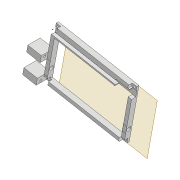
# Autodesk Inventor part: Rail_stage_y_v1
Saved by Autodesk Inventor 2020 (Build 240168000, 168)
## iProperties
Created: 2022-01-11
Part Number: Rail_stage_y_v1
Material: Generic
Document SubType Name: Modeling
Designer: CDT
Density: 1 g/cm^3
Appearance: Default
Author: CDT
Autodesk Inventor part; units mm, degrees
ref_plane "YZ Plane" through (0, 0, 0) normal (1, 0, 0) x (0, 1, 0)
ref_plane "XZ Plane" through (0, 0, 0) normal (0, 1, 0) x (-1, 0, 0)
ref_plane "XY Plane" through (0, 0, 0) normal (0, 0, 1) x (1, 0, 0)
ref_plane "Work Plane1" through (34.4543, -4.3418, 1.4) normal (0, 0, 1) x (0.9837071, -0.1797788, 0)
sketch "Sketch1" plane through (34.4543, -4.3418, 1.4) normal (0, 0, 1) x (0.9837071, -0.1797788, 0)
  line L0 (38.644, 42.2221) -> (-81.356, 42.2221)
  line L1 (-81.356, 42.2221) -> (-81.356, -37.7779)
  line L2 (-81.356, -37.7779) -> (38.644, -37.7779)
  line L3 (38.644, -37.7779) -> (38.644, 42.2221)
  circle A0 centre (35.644, 39.2221) radius 1.5
  circle A1 centre (35.644, -34.7779) radius 1.5
  circle A2 centre (-78.356, 39.2221) radius 1.5
  circle A3 centre (-78.356, -34.7779) radius 1.5
  line L4 (-76.356, 37.2221) -> (33.644, 37.2221)
  line L5 (33.644, 37.2221) -> (33.644, -32.7779)
  line L6 (33.644, -32.7779) -> (-76.356, -32.7779)
  line L7 (-76.356, -32.7779) -> (-76.356, 37.2221)
  line L8 (33.644, -11.7779) -> (32.644, -11.7779)
  line L9 (32.644, -11.7779) -> (32.644, -21.7779)
  line L10 (32.644, -21.7779) -> (33.644, -21.7779)
  line L11 (33.644, -21.7779) -> (33.644, -11.7779)
  point P0 (-34.6735, -1.9231)
  point P1 (33.644, -21.7779)
  dimension "d0" = 120
  dimension "d1" = 80
  dimension "d2" = 3
  dimension "d3" = 3
  dimension "d4" = 3
  dimension "d5" = 3
  dimension "d6" = 3
  dimension "d7" = 3
  dimension "d8" = 3
  dimension "d9" = 3
  dimension "d10" = 3
  dimension "d11" = 3
  dimension "d12" = 3
  dimension "d13" = 3
  dimension "d16" = 5
  dimension "d64" = 11
  dimension "d65" = 1
  dimension "d66" = 10
  constraints: 24 end point, 6 parallel, 4 centre point, 3 perpendicular, 2 horizontal, 1 point on line, 3 other
  measures "d0" distance of L2.end L1.end
  measures "d1" distance of L1.end L0.end
  measures "d2" diameter of A0
  measures "d3" diameter of A1
  measures "d4" diameter of A2
  measures "d5" diameter of A3
  measures "d6" distance from line of L0 A0.centre
  measures "d7" distance from line of L3 A0.centre
  measures "d8" distance from line of L2 A1.centre
  measures "d9" distance from line of L3 A1.centre
  measures "d10" distance from line of L1 A2.centre
  measures "d11" distance from line of L0 A2.centre
  measures "d12" distance from line of L1 A3.centre
  measures "d13" distance from line of L2 A3.centre
  measures "d16" distance between parallel lines of L0 L4
  measures "d64" distance between parallel lines of L6 L10
  measures "d65" distance between parallel lines of L5 L9
  measures "d66" distance between parallel lines of L10 L8
extrude "Extrusion1" add sketch "Sketch1" along normal blind 8 contours L3 L2 L1 L0 | L5 L10 L9 L8
sketch "Sketch3" plane through (34.4543, -4.3418, 9.4) normal (0, 0, 1) x (0.9837071, -0.1797788, 0)
  circle A0 centre (35.644, 39.2221) radius 1.5 projected
  circle A1 centre (35.644, -34.7779) radius 1.5 projected
  circle A2 centre (-78.356, 39.2221) radius 1.5 projected
  circle A3 centre (-78.356, -34.7779) radius 1.5 projected
  point P0 (-34.6735, -1.9231)
  point P1 (35.644, 39.2221)
  point P2 (35.644, -34.7779)
  point P3 (-78.356, 39.2221)
  point P4 (-78.356, -34.7779)
  constraints: 4 coincident
hole "Hole1" at (76.5689, 27.8333, 9.4) at (63.2653, -44.9611, 9.4) at (-35.5737, 48.328, 9.4) at (-48.8773, -24.4663, 9.4) direction (0, 0, -1) diameter 3.1 depth 8 tip angle 118 counterbore diameter 10 counterbore depth 5
sketch "Sketch6" plane through (34.4543, -4.3418, 1.4) normal (0, 0, -1) x (-0.9837071, 0.1797788, 0)
  line L0 (76.356, 37.2221) -> (-33.644, 37.2221) projected
  line L1 (76.356, 37.2221) -> (-33.644, 37.2221)
  line L2 (-33.644, 37.2221) -> (-33.644, 27.2221)
  line L3 (-33.644, 27.2221) -> (76.356, 27.2221)
  line L4 (76.356, 27.2221) -> (76.356, 37.2221)
  point P0 (34.6735, -1.9231)
  point P1 (-33.644, 37.2221)
  dimension "d43" = 110
  dimension "d44" = 10
  constraints: 8 end point, 2 parallel, 1 horizontal, 1 perpendicular
  measures "d43" distance of L3.end L2.end
  measures "d44" distance of L2.end L1.end
extrude "Extrusion5" add sketch "Sketch6" against normal up to surface (8 mm away)
sketch "Sketch7" plane through (34.4543, -4.3418, 9.4) normal (0, 0, 1) x (0.9837071, -0.1797788, 0)
  line L0 (38.644, 35.2221) -> (-81.356, 35.2221)
  line L1 (-81.356, 35.2221) -> (-81.356, 29.2221)
  line L2 (-81.356, 29.2221) -> (38.644, 29.2221)
  line L3 (38.644, 29.2221) -> (38.644, 35.2221)
  line L4 (31.644, 42.2221) -> (-74.356, 42.2221) projected
  line L5 (-81.356, 35.2221) -> (-81.356, -30.7779) projected
  line L6 (38.644, -30.7779) -> (38.644, 35.2221) projected
  point P0 (-34.6735, -1.9231)
  point P1 (38.644, 42.2221)
  point P2 (35.644, 42.2221)
  point P3 (-81.356, 42.2221)
  point P4 (-81.356, 39.2221)
  point P5 (38.644, -37.7779)
  point P6 (38.644, -34.7779)
  point P7 (-81.356, -37.7779)
  dimension "d47" = 6
  dimension "d48" = 7
  dimension "d49" = 0
  dimension "d50" = 0
  constraints: 8 end point, 2 parallel, 1 horizontal, 1 perpendicular
  measures "d47" distance of L1.end L0.end
  measures "d48" distance between parallel lines of L4 L0
  measures "d49" distance between parallel lines of L5 L1
  measures "d50" distance between parallel lines of L6 L3
extrude "Extrusion6" cut sketch "Sketch7" against normal blind 6 draft 10
sketch "Sketch8" plane through (65.6771, -48.4515, 1.4) normal (0.9837071, -0.1797788, 0) x (0, 0, -1)
  line L0 (-2, 74.5) -> (-9, 74.5)
  line L1 (-9, 74.5) -> (-9, 64.5)
  line L2 (-9, 64.5) -> (-2, 64.5)
  line L3 (-2, 64.5) -> (-2, 74.5)
  line L4 (0, 80) -> (-3, 80) projected
  line L5 (-2, 74.058) -> (-2, 65.942) projected
  point P0 (1.4, 35.8548)
  point P1 (-8, 80)
  dimension "d53" = 7
  dimension "d54" = 10
  dimension "d55" = 5.5
  dimension "d56" = 0
  constraints: 8 end point, 2 parallel, 1 horizontal, 1 perpendicular
  measures "d53" distance of L2.end L1.end
  measures "d54" distance of L1.end L0.end
  measures "d55" distance between parallel lines of L4 L0
  measures "d56" distance between parallel lines of L5 L3
extrude "Extrusion7" cut sketch "Sketch8" against normal blind 25
sketch "Sketch10" plane through (34.4543, -4.3418, 1.4) normal (0, 0, -1) x (-0.9837071, 0.1797788, 0)
  line L0 (81.356, 4.2221) -> (101.356, 4.2221)
  line L1 (101.356, 4.2221) -> (101.356, -5.7779)
  line L2 (101.356, -5.7779) -> (81.356, -5.7779)
  line L3 (81.356, -5.7779) -> (81.356, 4.2221)
  line L4 (81.356, -27.7779) -> (101.356, -27.7779)
  line L5 (101.356, -27.7779) -> (101.356, -37.7779)
  line L6 (101.356, -37.7779) -> (81.356, -37.7779)
  line L7 (81.356, -37.7779) -> (81.356, -27.7779)
  line L8 (81.356, 42.2221) -> (81.356, -37.7779) projected
  line L9 (81.356, -37.7779) -> (-38.644, -37.7779) projected
  point P0 (34.6735, -1.9231)
  dimension "d67" = 0
  dimension "d68" = 10
  dimension "d69" = 20
  dimension "d70" = 22
  dimension "d71" = 0
  dimension "d72" = 10
  dimension "d73" = 0
  dimension "d74" = 20
  constraints: 16 end point, 4 parallel, 2 horizontal, 2 perpendicular
  measures "d67" distance between parallel lines of L8 L3
  measures "d68" distance between parallel lines of L0 L2
  measures "d69" distance between parallel lines of L1 L3
  measures "d70" distance between parallel lines of L4 L2
  measures "d71" distance between parallel lines of L9 L6
  measures "d72" distance between parallel lines of L6 L4
  measures "d73" distance between parallel lines of L8 L7
  measures "d74" distance between parallel lines of L5 L7
extrude "Extrusion9" add sketch "Sketch10" against normal blind 18
sketch "Sketch12" plane through (34.4543, -4.3418, 9.4) normal (0, 0, 1) x (0.9837071, -0.1797788, 0)
  line L0 (-76.356, -30.1953) -> (-76.356, 27.2221) projected
  line L1 (-76.356, -5.7779) -> (-81.356, -5.7779)
  line L2 (-81.356, -5.7779) -> (-81.356, -27.7779)
  line L3 (-81.356, -27.7779) -> (-76.356, -27.7779)
  line L4 (-76.356, -27.7779) -> (-76.356, -5.7779)
  line L5 (-81.356, -5.7779) -> (-81.356, -27.7779) projected
  line L6 (-74.356, -37.7779) -> (31.644, -37.7779) projected
  line L7 (-101.356, -5.7779) -> (-81.356, -5.7779) projected
  line L8 (32.644, -11.7779) -> (32.644, -21.7779) projected
  line L9 (32.644, -11.7779) -> (38.644, -11.7779)
  line L10 (38.644, -11.7779) -> (38.644, -21.7779)
  line L11 (38.644, -21.7779) -> (32.644, -21.7779)
  line L12 (32.644, -21.7779) -> (32.644, -11.7779)
  line L13 (38.644, -30.7779) -> (38.644, 26.7221) projected
  line L14 (32.644, -21.7779) -> (33.644, -21.7779) projected
  point P0 (-34.6735, -1.9231)
  point P1 (-78.356, -37.7779)
  point P2 (35.644, -37.7779)
  point P3 (-76.356, -27.7779)
  point P4 (38.644, -34.7779)
  point P5 (32.644, -21.7779)
  point P6 (-81.356, -37.7779)
  point P7 (-80.606, -37.7779)
  point P8 (38.644, -37.7779)
  dimension "d78" = 0
  dimension "d79" = 10
  dimension "d80" = 0
  dimension "d88" = 0
  dimension "d89" = 0
  constraints: 16 end point, 4 parallel, 2 horizontal, 2 perpendicular, 1 point on line
  measures "d78" distance between parallel lines of L5 L2
  measures "d79" distance between parallel lines of L6 L3
  measures "d80" distance between parallel lines of L7 L1
  measures "d88" distance between parallel lines of L13 L10
  measures "d89" distance between parallel lines of L14 L11
extrude "Extrusion10" add sketch "Sketch12" along normal blind 0.0001
sketch "Sketch13" plane through (-50.57, -17.041, 1.4) normal (-0.9837071, 0.1797788, 0) x (0, 0, 1)
  circle A0 centre (4.2501, 10.5) radius 3.1
  line L0 (0, -10) -> (18, -10) projected
  line L1 (8.0001, 22) -> (8.0001, 0) projected
  point P0 (-1.4, 25.8548)
  dimension "d83" = 6.2
  dimension "d84" = 20.5
  dimension "d85" = 3.75
  constraints: 1 centre point
  measures "d83" diameter of A0
  measures "d84" distance from line of L0 A0.centre
  measures "d85" distance from line of L1 A0.centre
extrude "Extrusion11" cut sketch "Sketch13" against normal through all
sketch "Sketch14" plane through (-66.289, 8.1961, 1.4) normal (-0.9837071, 0.1797788, 0) x (0, 0, 1)
  circle A0 centre (12.2501, 6) radius 1.75
  circle A1 centre (12.2501, -29) radius 1.75
  circle A2 centre (4.2501, -11.5) radius 3.1 projected
  point P0 (-1.4, 3.8548)
  dimension "d90" = 3.5
  dimension "d91" = 3.5
  dimension "d92" = 17.5
  dimension "d93" = 8
  dimension "d94" = 8
  dimension "d95" = 17.5
  constraints: 2 centre point
  measures "d90" diameter of A0
  measures "d91" diameter of A1
  measures "d92" vertical distance of A1.centre A2.centre
  measures "d93" horizontal distance of A2.centre A1.centre
  measures "d94" horizontal distance of A2.centre A0.centre
  measures "d95" vertical distance of A2.centre A0.centre
extrude "Extrusion12" cut sketch "Sketch14" against normal through all contours A0 | A1
chamfer "Chamfer1" distance 1 angle 45 1 edges at (63.5502, -26.715, 9.4001)
sketch "Sketch16" plane through (34.4543, -4.3418, 1.4) normal (0, 0, -1) x (-0.9837071, 0.1797788, 0)
  circle A0 centre (36.356, 32.7221) radius 1.5
  circle A1 centre (61.356, 32.7221) radius 1.5
  circle A2 centre (11.356, 32.7221) radius 1.5
  line L0 (81.356, 42.2221) -> (81.356, 4.2221) projected
  line L1 (-33.644, 27.2221) -> (76.356, 27.2221) projected
  point P0 (34.6735, -1.9231)
  dimension "d112" = 3
  dimension "d113" = 3
  dimension "d114" = 3
  dimension "d115" = 20
  dimension "d116" = 5.5
  dimension "d117" = 25
  dimension "d118" = 5.5
  dimension "d119" = 25
  dimension "d120" = 5.5
  constraints: 3 centre point
  measures "d112" diameter of A0
  measures "d113" diameter of A1
  measures "d114" diameter of A2
  measures "d115" distance from line of L0 A1.centre
  measures "d116" distance from line of L1 A1.centre
  measures "d117" distance of A1.centre A0.centre
  measures "d118" distance from line of L1 A0.centre
  measures "d119" distance of A0.centre A2.centre
  measures "d120" distance from line of L1 A2.centre
extrude "Extrusion14" cut sketch "Sketch16" against normal through all
equation "\"d72\" = d68"
equation "\"d74\" = d69"
equation "\"d94\" = d93"
equation "\"d95\" = d92"
equation "\"d118\" = d116"
equation "\"d120\" = d118"
body "Solid1"
